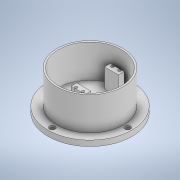
# Autodesk Inventor part: Base Part
Saved by Autodesk Inventor 2022 (Build 260153000, 153)
## iProperties
Created: 2022-02-03
Part Number: Base Part
Material: Generic
Document SubType Name: Modeling
Designer: Alexa
Density: 1 g/cm^3
Appearance: Default
Author: Alexa
Autodesk Inventor part; units mm, degrees
ref_plane "YZ Plane" through (0, 0, 0) normal (1, 0, 0) x (0, 1, 0)
ref_plane "XZ Plane" through (0, 0, 0) normal (0, 1, 0) x (-1, 0, 0)
ref_plane "XY Plane" through (0, 0, 0) normal (0, 0, 1) x (1, 0, 0)
sketch "Sketch1" plane through (0, 0, 0) normal (0, 1, 0) x (-1, 0, 0)
  circle A0 centre (0, 0) radius 60
  dimension "d0" = 120
  constraints: 1 centre point, 1 coincident
  measures "d0" diameter of A0
extrude "Extrusion1" add sketch "Sketch1" along normal blind 8
sketch "Sketch2" plane through (0, 8, 0) normal (0, 1, 0) x (1, 0, 0)
  circle A0 centre (-54, 0) radius 4
  circle A1 centre (-54, 0) radius 2.5
  circle A2 centre (0, -54) radius 4
  circle A3 centre (0, -54) radius 2.5
  circle A4 centre (54, 0) radius 4
  circle A5 centre (54, 0) radius 2.5
  circle A6 centre (0, 54) radius 4
  circle A7 centre (0, 54) radius 2.5
  point P0 (0, 0)
  dimension "d3" = 8
  dimension "d4" = 5
  dimension "d5" = 8
  dimension "d6" = 5
  dimension "d7" = 8
  dimension "d8" = 5
  dimension "d9" = 8
  dimension "d10" = 5
  constraints: 8 centre point, 4 coincident
  measures "d3" diameter of A0
  measures "d4" diameter of A1
  measures "d5" diameter of A2
  measures "d6" diameter of A3
  measures "d7" diameter of A4
  measures "d8" diameter of A5
  measures "d9" diameter of A6
  measures "d10" diameter of A7
extrude "Extrusion2" cut sketch "Sketch2" against normal blind 8 contours A1 | A3 | A5 | A7
sketch "Sketch3" plane through (0, 8, 0) normal (0, 1, 0) x (1, 0, 0)
  circle A0 centre (-54, 0) radius 2.5 projected
  circle A1 centre (-54, 0) radius 4
  circle A2 centre (-54, 0) radius 2.5
  circle A3 centre (0, 54) radius 2.5 projected
  circle A4 centre (0, 54) radius 4
  circle A5 centre (0, 54) radius 2.5
  circle A6 centre (54, 0) radius 2.5 projected
  circle A7 centre (54, 0) radius 4
  circle A8 centre (54, 0) radius 2.5
  circle A9 centre (0, -54) radius 4
  circle A10 centre (0, -54) radius 2.5
  point P0 (0, 0)
  dimension "d13" = 8
  dimension "d14" = 8
  dimension "d15" = 5
  dimension "d16" = 8
  dimension "d17" = 5
  dimension "d18" = 8
  constraints: 8 centre point, 7 coincident
  measures "d13" diameter of A1
  measures "d14" diameter of A4
  measures "d15" diameter of A5
  measures "d16" diameter of A7
  measures "d17" diameter of A8
  measures "d18" diameter of A9
extrude "Extrusion3" cut sketch "Sketch3" against normal blind 3
sketch "Sketch4" plane through (0, 8, 0) normal (0, 1, 0) x (1, 0, 0)
  circle A0 centre (0, 0) radius 47.5
  circle A1 centre (0, 0) radius 45
  line L0 (0, 0) -> (-10, 0)
  line L1 (-10, 0) -> (-10, -9)
  line L2 (-10, -9) -> (0, -9)
  line L3 (0, -9) -> (0, 0)
  line L4 (0, -9) -> (10, -9)
  line L5 (10, -9) -> (10, 0)
  line L6 (10, 0) -> (0, 0)
  line L7 (0, 0) -> (0, -9)
  line L8 (-10, -9) -> (10, -9)
  line L9 (10, -9) -> (10, -16)
  line L10 (10, -16) -> (-10, -16)
  line L11 (-10, -16) -> (-10, -9)
  dimension "d21" = 95
  dimension "d22" = 90
  dimension "d23" = 10
  dimension "d24" = 9
  dimension "d25" = 10
  dimension "d26" = 7
  constraints: 24 end point, 6 parallel, 3 horizontal, 3 perpendicular, 2 centre point, 2 coincident, 1 point on line
  measures "d21" diameter of A0
  measures "d22" diameter of A1
  measures "d23" distance of L2.end L1.end
  measures "d24" distance of L1.end L0.end
  measures "d25" distance of L6.end L5.end
  measures "d26" distance of L8.end L9.end
extrude "Extrusion4" add sketch "Sketch4" along normal blind 47.5 contours A0
sketch "Sketch5" plane through (0, 8, 0) normal (0, 1, 0) x (1, 0, 0)
  line L0 (0, 0) -> (-10, 0)
  line L1 (-10, 0) -> (-10, -9)
  line L2 (-10, -9) -> (0, -9)
  line L3 (0, -9) -> (0, 0)
  line L4 (-10, -9) -> (10, -9)
  line L5 (10, -9) -> (10, -16)
  line L6 (10, -16) -> (-10, -16)
  line L7 (-10, -16) -> (-10, -9)
  line L8 (-10, -9) -> (10, -9)
  line L9 (10, -9) -> (10, 31)
  line L10 (10, 31) -> (-10, 31)
  line L11 (-10, 31) -> (-10, -9)
  line L12 (-10, 31) -> (-2, 31)
  line L13 (-2, 31) -> (-2, 38.36)
  line L14 (-2, 38.36) -> (-10, 38.36)
  line L15 (-10, 38.36) -> (-10, 31)
  line L16 (-10, 31) -> (10, 31)
  line L17 (10, 31) -> (10, 39)
  line L18 (10, 39) -> (-10, 39)
  line L19 (-10, 39) -> (-10, 31)
  line L20 (-10, -9) -> (10, -9)
  line L21 (10, -9) -> (10, -17)
  line L22 (10, -17) -> (-10, -17)
  line L23 (-10, -17) -> (-10, -9)
  dimension "d29" = 10
  dimension "d30" = 9
  dimension "d31" = 20
  dimension "d32" = 7
  dimension "d33" = 40
  dimension "d34" = 8
  dimension "d35" = 8
  dimension "d36" = 8
  constraints: 48 end point, 12 parallel, 6 horizontal, 6 perpendicular, 3 point on line
  measures "d29" distance of L2.end L1.end
  measures "d30" distance of L1.end L0.end
  measures "d31" distance of L5.end L6.end
  measures "d32" distance of L4.end L5.end
  measures "d33" distance of L9.end L8.end
  measures "d34" distance of L14.end L13.end
  measures "d35" distance of L17.end L16.end
  measures "d36" distance of L20.end L21.end
extrude "Extrusion5" add sketch "Sketch5" along normal blind 28 contours L4 L5 L6 L7 L2 | L15 L14 L13 L10 | L6 L21 L22 L23 | L13 L14 L19 L18 L17 L10
sketch "Sketch6" plane through (0, 36, 0) normal (0, 1, 0) x (1, 0, 0)
  line L0 (10, -17) -> (-10, -17) projected
  line L1 (-10, -9) -> (10, -9) projected
  line L2 (0, -17) -> (-4, -17)
  line L3 (-4, -17) -> (-4, -9)
  line L4 (-4, -9) -> (0, -9)
  line L5 (0, -9) -> (0, -17)
  line L6 (0, -17) -> (4, -17)
  line L7 (4, -17) -> (4, -9)
  line L8 (4, -9) -> (0, -9)
  line L9 (0, -9) -> (0, -17)
  point P0 (0, 0)
  dimension "d39" = 4
  dimension "d40" = 4
  constraints: 16 end point, 4 parallel, 2 horizontal, 2 perpendicular, 2 point on line, 1 midpoint
  measures "d39" distance of L3.end L4.end
  measures "d40" distance of L8.end L7.end
extrude "Extrusion6" cut sketch "Sketch6" against normal blind 28
sketch "Sketch7" plane through (0, 36, 0) normal (0, 1, 0) x (1, 0, 0)
  line L0 (-10, -17) -> (-4, -17) projected
  line L1 (4, -9) -> (10, -9) projected
  line L2 (-4, -17) -> (4, -17)
  line L3 (4, -17) -> (4, -9)
  line L4 (4, -9) -> (-4, -9)
  line L5 (-4, -9) -> (-4, -17)
  point P0 (0, 0)
  constraints: 8 end point, 2 parallel, 1 horizontal, 1 perpendicular
extrude "Extrusion7" add sketch "Sketch7" against normal blind 22
sketch "Sketch8" plane through (0, 36, 0) normal (0, 1, 0) x (1, 0, 0)
  line L0 (-4, -17) -> (-10, -17) projected
  line L1 (10, -17) -> (10, -9) projected
  line L2 (-10, -17) -> (10, -17)
  line L3 (10, -17) -> (10, -15)
  line L4 (10, -15) -> (-10, -15)
  line L5 (-10, -15) -> (-10, -17)
  line L6 (-4, -9) -> (4, -9) projected
  line L7 (0, -9) -> (-5, -9)
  line L8 (-5, -9) -> (-5, -17)
  line L9 (-5, -17) -> (0, -17)
  line L10 (0, -17) -> (0, -9)
  line L11 (-10, -17) -> (10, -17) projected
  line L12 (0, -9) -> (5, -9)
  line L13 (5, -9) -> (5, -17)
  line L14 (5, -17) -> (0, -17)
  line L15 (0, -17) -> (0, -9)
  circle A0 centre (-5, -15) radius 2
  circle A1 centre (5, -15) radius 2
  line L16 (-10, 31) -> (-10, 39) projected
  line L17 (10, 39) -> (10, 31) projected
  line L18 (-10, 39) -> (10, 39)
  line L19 (10, 39) -> (10, 37)
  line L20 (10, 37) -> (-10, 37)
  line L21 (-10, 37) -> (-10, 39)
  line L22 (10, 31) -> (-10, 31) projected
  line L23 (-10, 39) -> (10, 39) projected
  line L24 (0, 31) -> (-5, 31)
  line L25 (-5, 31) -> (-5, 39)
  line L26 (-5, 39) -> (0, 39)
  line L27 (0, 39) -> (0, 31)
  line L28 (0, 31) -> (5, 31)
  line L29 (5, 31) -> (5, 39)
  line L30 (5, 39) -> (0, 39)
  line L31 (0, 39) -> (0, 31)
  circle A2 centre (-5, 37) radius 2
  circle A3 centre (5, 37) radius 2
  point P0 (0, 0)
  dimension "d45" = 2
  dimension "d46" = 5
  dimension "d47" = 5
  dimension "d48" = 4
  dimension "d49" = 4
  dimension "d50" = 2
  dimension "d51" = 4
  dimension "d52" = 4
  constraints: 48 end point, 14 point on line, 12 parallel, 6 horizontal, 6 perpendicular, 4 centre point, 2 midpoint
  measures "d45" distance of L3.end L2.end
  measures "d46" distance of L9.end L8.end
  measures "d47" distance of L13.end L14.end
  measures "d48" diameter of A0
  measures "d49" diameter of A1
  measures "d50" distance of L18.end L19.end
  measures "d51" diameter of A2
  measures "d52" diameter of A3
extrude "Extrusion8" cut sketch "Sketch8" against normal blind 10 contours A0 L4 L8 | L8 L4 A0 | L8 A0 L4 | L4 A0 L8 | A1 L4 L13 | L13 L4 A1 | L13 A1 L4 | L4 A1 L13 | A2 L25 L20 | L20 L25 A2 | L25 L20 A2 | A2 L20 L25 | A3 L20 L29 | L29 L20 A3 | A3 L29 L20 | A3 L20 L29
body "Solid1"
